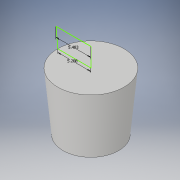
# Autodesk Inventor part: smokestack dimentions
Saved by Autodesk Inventor 2017 (Build 210142000, 142)
## iProperties
Created: 2017-12-27
Part Number: smokestack dimentions
Material: Generic
Document SubType Name: Modeling
Designer: Micah
Density: 1 g/cm^3
Appearance: Default
Author: Micah
Autodesk Inventor part; units mm, degrees
ref_plane "YZ Plane" through (0, 0, 0) normal (1, 0, 0) x (0, 1, 0)
ref_plane "XZ Plane" through (0, 0, 0) normal (0, 1, 0) x (-1, 0, 0)
ref_plane "XY Plane" through (0, 0, 0) normal (0, 0, 1) x (1, 0, 0)
sketch "Sketch2" plane through (0, 0, 0) normal (0, 0, 1) x (1, 0, 0)
  line L0 (110.7567, 0) -> (110.7567, 304.8)
  line L1 (110.7567, 304.8) -> (-28.4988, 304.8)
  line L2 (-28.4988, 304.8) -> (0, 0)
  line L3 (110.7567, 230.3409) -> (-21.5369, 230.3409)
  line L4 (0, 0) -> (110.7567, 0)
  dimension "d2" = 139.2555
  dimension "d9" = 132.2936
  constraints: 10 end point, 2 horizontal, 2 point on line, 1 vertical
  measures "d2" distance of L0.end L1.end
  measures "d9" distance of L3.start L3.end
revolve "Revolution2" add sketch "Sketch2" angle 360 about axis through (110.7567, 0, 0) along (0, 1, 0) contours L4 L2 L3 L0
body "Solid2"
